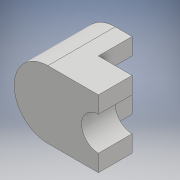
# Autodesk Inventor part: 29
Saved by Autodesk Inventor 2017 (Build 210142000, 142)
## iProperties
Part Number: 29
Material: 一般
Document SubType Name: Modeling
Designer: Brian
Density: 1 g/cm^3
Appearance: 預設
Author: Brian
Autodesk Inventor part; units mm, degrees
ref_plane "YZ Plane" through (0, 0, 0) normal (1, 0, 0) x (0, 1, 0)
ref_plane "XZ Plane" through (0, 0, 0) normal (0, 1, 0) x (-1, 0, 0)
ref_plane "XY Plane" through (0, 0, 0) normal (0, 0, 1) x (1, 0, 0)
sketch "草圖1" plane through (0, 0, 0) normal (0, 1, 0) x (-1, 0, 0)
  line L0 (0, 0) -> (-50, 0)
  line L1 (-50, 0) -> (-50, -40)
  line L2 (-50, -40) -> (0, -40)
  line L3 (0, -40) -> (0, 0)
  dimension "d0" = 50
  dimension "d1" = 40
  constraints: 8 end point, 2 parallel, 1 horizontal, 1 perpendicular
  measures "d0" distance of L1.end L2.end
  measures "d1" distance of L2.end L0.start
extrude "擠出1" add sketch "草圖1" along normal blind 20
sketch "草圖2" plane through (0, 20, 0) normal (0, 1, 0) x (1, 0, 0)
  line L0 (50, 40) -> (0, 40) projected
  line L1 (0, 0) -> (50, 0) projected
  line L2 (0, 40) -> (30, 40)
  line L3 (30, 40) -> (30, 0)
  line L4 (30, 0) -> (0, 0)
  line L5 (0, 0) -> (0, 40)
  dimension "d4" = 30
  constraints: 8 end point, 2 parallel, 1 horizontal, 1 perpendicular, 1 point on line
  measures "d4" distance between parallel lines of L5 L3
extrude "擠出2" add sketch "草圖2" along normal blind 20
fillet "圓角1" radius 20 2 edges at (0, 20, 0) (0, 20, -40)
sketch "草圖3" plane through (0, 40, 0) normal (0, 1, 0) x (1, 0, 0)
  arc A0 (20, 40) -> (20, 0) centre (20, 20) ccw projected
  line L0 (20, 0) -> (30, 0) projected
  line L1 (30, 0) -> (30, 40) projected
  line L2 (30, 40) -> (20, 40) projected
  arc A1 (20, 30) -> (20, 10) centre (20, 20) ccw
  line L3 (20, 30) -> (20, 30)
  line L4 (20, 30) -> (20, 10)
  line L5 (20, 10) -> (20, 10)
  line L6 (20, 30) -> (39.9509, 30)
  line L7 (39.9509, 30) -> (39.9509, 10)
  line L8 (39.9509, 10) -> (20, 10)
  line L9 (20, 10) -> (20, 30)
  point P0 (0, 0)
  dimension "d8" = 20
  constraints: 14 end point, 2 parallel, 2 point on circle, 1 centre point, 1 horizontal, 1 perpendicular, 3 other
  measures "d8" distance of L3.end L4.end
extrude "擠出3" cut sketch "草圖3" against normal blind 20 contours L6 L7 L8 L1 | L1 L8 L4 L6 | L4 A1
sketch "草圖4" plane through (0, 20, 0) normal (0, 1, 0) x (1, 0, 0)
  line L0 (50, 0) -> (50, 40) projected
  circle A0 centre (50, 20) radius 10
  point P0 (0, 0)
  dimension "d11" = 20
  constraints: 1 centre point, 1 midpoint
  measures "d11" diameter of A0
extrude "擠出4" cut sketch "草圖4" against normal blind 20
